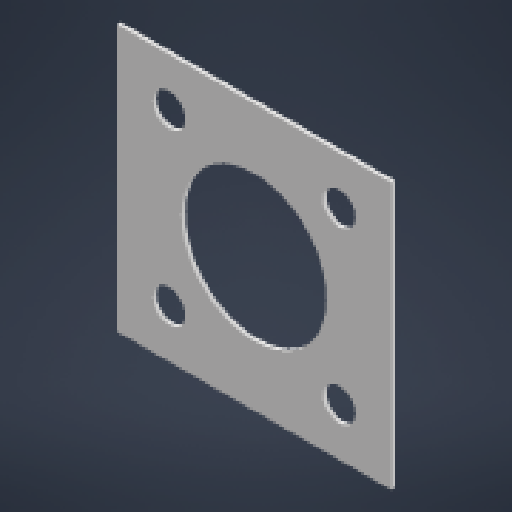
# Autodesk Inventor part: LoadCellMountFrame
Saved by Autodesk Inventor 2024 (Build 280153000, 153)
## iProperties
Created: 2025-02-08
Part Number: LoadCellMountFrame
Material: Generic
Document SubType Name: Sheet Metal
Designer: Tommy Rohmann
Density: 1 g/cm^3
Sheet Metal Rule: Default
Appearance: Default
Author: Tommy Rohmann
Autodesk Inventor part; units mm, degrees
ref_plane "YZ Plane" through (0, 0, 0) normal (1, 0, 0) x (0, 1, 0)
ref_plane "XZ Plane" through (0, 0, 0) normal (0, 1, 0) x (-1, 0, 0)
ref_plane "XY Plane" through (0, 0, 0) normal (0, 0, 1) x (1, 0, 0)
sketch "LoadCellMountFrame" plane through (0, 0, 0) normal (0, 0, 1) x (1, 0, 0)
  line L0 (410.7305, -425.004) -> (440.9764, -425.004)
  circle A0 centre (477.6334, -420.0135) radius 12.7
  line L1 (518.6805, -382.1415) -> (410.7305, -382.1415)
  line L2 (410.7305, -382.1415) -> (410.7305, -486.9165)
  line L3 (410.7305, -486.9165) -> (518.6805, -486.9165)
  line L4 (518.6805, -486.9165) -> (518.6805, -382.1415)
  point P0 (455.0461, -430.4944)
  dimension "d446" = 25.4
  measures "d446" diameter of A0
derived "LAYOUT.ipt"
sketch "Sketch1" plane through (0, 0, 0) normal (0, 0, 1) x (1, 0, 0)
  circle A0 centre (410.7305, -486.9165) radius 57.15
  line L0 (410.7305, -425.004) -> (440.9764, -425.004)
  circle A1 centre (477.6334, -420.0135) radius 12.7
  line L1 (518.6805, -382.1415) -> (410.7305, -382.1415)
  line L2 (410.7305, -382.1415) -> (410.7305, -486.9165)
  line L3 (410.7305, -486.9165) -> (518.6805, -486.9165)
  line L4 (518.6805, -486.9165) -> (518.6805, -382.1415)
  point P0 (410.7305, -429.7665)
  point P1 (467.8805, -486.9165)
  dimension "d1" = 114.3
  measures "d1" diameter of A0
extrude "Plate1" add sketch "Sketch1" along normal blind 3.048 contours A0 L2 L1 L4 L3
mirror "Mirror1" about plane through (518.6805, -486.9165, 0) normal (0, -1, 0)
mirror "Mirror2" about plane through (410.7305, -544.0665, 0) normal (-1, 0, 0)
equation "\"d2\" = Thickness"
equation "\"BendRadius\" = Thickness"
equation "\"BendReliefWidth\" = Thickness"
equation "\"BendReliefDepth\" = 0.5 * Thickness"
equation "\"CornerReliefSize\" = 4 * Thickness"
equation "\"MinimumRemnant\" = 2 * Thickness"
equation "\"TransitionRadius\" = BendRadius"
equation "\"JacobiRadiusSize\" = BendRadius"
equation "\"GapSize\" = Thickness"
equation "\"Thickness\" = 3.048"
body "Solid1"
